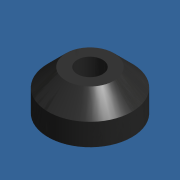
# Autodesk Inventor part: Shouder_spanner_Scheibe
Saved by Autodesk Inventor 2016 (Build 200138000, 138)
## iProperties
Created: 2015-02-18
Part Number: Shouder_spanner_Scheibe
Material: ABS-Kunststoff - Schwarz
Document SubType Name: Modeling
Designer: 4ndreas
Density: 1.06 g/cm^3
Appearance: Glatt - weiß(2)
Author: 4ndreas
Autodesk Inventor part; units mm, degrees
ref_plane "YZ Plane" through (0, 0, 0) normal (1, 0, 0) x (0, 1, 0)
ref_plane "XZ Plane" through (0, 0, 0) normal (0, 1, 0) x (-1, 0, 0)
sketch "Skizze1" plane through (0, 0, 0) normal (0, 0, 1) x (1, 0, 0)
  circle A0 centre (18.6329, -33.6593) radius 2.1
  circle A1 centre (18.6329, -33.6593) radius 7
  point P0 (0, 0)
  dimension "d0" = 4.2
  dimension "d1" = 14
  constraints: 2 centre point, 2 coincident, 1 other
  measures "d0" diameter of A0
  measures "d1" diameter of A1
ref_plane "Arbeitsebene1" through (14.6329, -37.6593, 6.675) normal (0, 0, -1) x (0, 1, 0)
extrude "Extrusion1" add sketch "Skizze1" along normal up to surface (6.675 mm away)
chamfer "Fase1" distance 3 angle 45 1 edges at (11.6329, -33.6593, 6.675)
